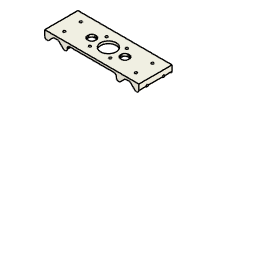
CHASSI_Pcb_SHELF (Autodesk Fusion 360 design; units mm, degrees)
Autodesk Fusion 360 part; units mm, degrees
note: some values were not read from the file. Set by a fixed rule: which sketch regions a step uses.
sketch "Sketch1" plane through (0, 21.15, 0) normal (0, 1, 0) x (-1, 0, 0)
  line L0 (-10, -11.15) -> (-10, 92)
  line L1 (-10, 92) -> (-12.5, 92)
  line L2 (-12.5, 92) -> (-12.5, -11.15)
  line L3 (-12.5, -11.15) -> (-10, -11.15)
  line L4 (112.5, -11.15) -> (112.5, 92)
  line L5 (112.5, 92) -> (110, 92)
  line L6 (110, 92) -> (110, -11.15)
  line L7 (110, -11.15) -> (112.5, -11.15)
  line L8 (81.2426, 69) -> (18.7574, 69)
  line L9 (18.7574, 69) -> (7.3788, 57.6216)
  line L10 (7.3788, 57.6216) -> (1.3788, 57.6216)
  line L11 (1.3788, 57.6216) -> (-10, 69.0007)
  line L12 (-10, 69.0007) -> (-10, 36.0007)
  line L13 (-10, 36.0007) -> (20, 66)
  line L14 (20, 66) -> (80, 66)
  line L15 (80, 66) -> (110, 36)
  line L16 (110, 36) -> (110, 69)
  line L17 (110, 69) -> (98.6213, 57.6213)
  line L18 (98.6213, 57.6213) -> (92.6213, 57.6213)
  line L19 (92.6213, 57.6213) -> (81.2426, 69)
  line L20 (50, 69) -> (50, 89) construction
  line L21 (-10, 92) -> (110, 92)
  line L22 (1.3788, 57.6216) -> (-10, 69.0007)
  line L23 (7.3788, 57.6216) -> (1.3788, 57.6216)
  line L24 (18.7574, 69) -> (7.3788, 57.6216)
  line L25 (4.3788, 57.6216) -> (4.3788, 89) construction
  line L26 (18.7574, 69) -> (7.3788, 57.6216)
  line L27 (7.3788, 57.6216) -> (1.3788, 57.6216)
  line L28 (1.3788, 57.6216) -> (-10, 69.0007)
  line L29 (7.3788, 57.6216) -> (18.7574, 69)
  line L30 (18.7574, 69) -> (24.7574, 69)
  line L31 (24.7574, 69) -> (36.1361, 57.621)
  line L32 (-9.9999, 77.6216) -> (1.3788, 89)
  line L33 (1.3788, 89) -> (7.3788, 89)
  line L34 (7.3788, 89) -> (18.7575, 77.621)
  line L35 (-10, 92) -> (-9.9999, 77.6216)
  line L36 (18.7575, 77.621) -> (18.7575, 89)
  line L37 (4.3788, 89) -> (7.3788, 89)
  line L38 (92.6213, 89) -> (81.2425, 77.621)
  line L39 (98.6213, 89) -> (92.6213, 89)
  line L40 (109.9999, 77.6216) -> (98.6213, 89)
  line L41 (81.2425, 77.621) -> (81.2425, 89)
  line L42 (18.7575, 89) -> (81.2425, 89)
  line L43 (92.6213, 89) -> (98.6213, 89)
  line L44 (110, 92) -> (109.9999, 77.6216)
  dimension "d70" = 20
  constraint midpoint L8 L20.start
  constraint perpendicular L8 L20
  constraint perpendicular L6 L37
  constraint midpoint L10 L25.start
  constraint perpendicular L25 L37
  constraint coincident L36.end L37
  constraint perpendicular L36 L37
  constraint collinear L37 L42
  constraint symmetric L20 L32.end L39.start
  constraint symmetric L20 L34.end L38.end
  constraint symmetric L20 L33.end L38.start
  constraint symmetric L20 L32.start L40.start
  constraint symmetric L20 L36.end L41.end
  constraint collinear L42 L43
  constraint coincident L5.end L6.start
  measures "d70" distance of L20.start L20.end
extrude "Extrude1" add sketch "Sketch1" against normal blind 42.3 contours L0 L6 L21 L32 L33 L34 L35 L36 L37 L38 L39 L40 L41 L42 L43 L44
sketch "Sketch2" plane through (9.9991, 0, -0.0001) normal (1, 0, -0.00001) x (0, 1, 0)
  line L0 (21.15, 77.6217) -> (21.15, 92.0001)
  line L1 (21.15, 92.0001) -> (-21.15, 92.0001)
  line L2 (-21.15, 92.0001) -> (-21.15, 77.6217)
  line L3 (-21.15, 77.6217) -> (21.15, 77.6217)
  line L4 (-21.15, 84.8109) -> (0, 84.8109) construction
  line L5 (0, 84.8109) -> (21.15, 84.8109) construction
  circle A0 centre (-10.575, 84.8109) radius 1.5
  circle A1 centre (10.575, 84.8109) radius 1.5
  dimension "d74" = 3
  dimension "d75" = 3
  constraint midpoint L2 L4.start
  constraint perpendicular L2 L4
  constraint midpoint L0 L5.end
  constraint perpendicular L0 L5
  constraint midpoint L4 A0.centre
  constraint midpoint L5 A1.centre
  measures "d74" diameter of A0
  measures "d75" diameter of A1
extrude "Extrude2" cut sketch "Sketch2" against normal blind 4 contours A0 | A1
sketch "Sketch4" plane through (-109.9992, 0, -0.0009) normal (-1, 0, -0.000008) x (0, -1, 0)
  line L0 (-21.15, 92.0009) -> (-21.15, 77.6226)
  line L1 (-21.15, 77.6226) -> (21.15, 77.6226)
  line L2 (21.15, 77.6226) -> (21.15, 92.0009)
  line L3 (21.15, 92.0009) -> (-21.15, 92.0009)
  ellipse E0 centre (10.575, 84.8107) end of major axis (9.075, 84.8107) minor radius 1.5
  ellipse E1 centre (-10.575, 84.8107) end of major axis (-12.075, 84.8107) minor radius 1.5
  ellipse E2 centre (0, 60.7499) end of major axis (-1.5, 60.7499) minor radius 1.5
  ellipse E3 centre (-10.575, 52.4999) end of major axis (-12.075, 52.4999) minor radius 1.5
  ellipse E4 centre (10.575, 52.4999) end of major axis (9.075, 52.4999) minor radius 1.5
  ellipse E5 centre (0, 44.2499) end of major axis (-1.5, 44.2499) minor radius 1.5
  ellipse E6 centre (15.5, 15.4999) end of major axis (14, 15.4999) minor radius 1.5
  ellipse E7 centre (-15.5, 15.4999) end of major axis (-17, 15.4999) minor radius 1.5
  ellipse E8 centre (-15.5, -15.5001) end of major axis (-17, -15.5001) minor radius 1.5
  ellipse E9 centre (15.5, -15.5001) end of major axis (14, -15.5001) minor radius 1.5
  ellipse E10 centre (0, -0.0001) end of major axis (-11, -0.0001) minor radius 11
  line L4 (21.15, 91.9999) -> (21.15, -11.1501)
  ellipse E11 centre (11.15, -11.1501) end of major axis (21.15, -11.1501) minor radius 10 (11.15, -21.1501) -> (21.15, -11.1501) ccw
  line L5 (11.15, -21.1501) -> (-11.15, -21.1501)
  ellipse E12 centre (-11.15, -11.1501) end of major axis (-21.15, -11.1501) minor radius 10 (-21.15, -11.1501) -> (-11.15, -21.1501) ccw
  line L6 (-21.15, -11.1501) -> (-21.15, 91.9999)
  line L7 (-21.15, 91.9999) -> (21.15, 91.9999)
extrude "Extrude4" cut sketch "Sketch4" against normal blind 4 contours E0 | E1
sketch "Sketch5" plane through (0, 0, 92) normal (0, 0, 1) x (-1, 0, 0)
  line L0 (-10, -21.15) -> (110, -21.15)
  line L1 (110, -21.15) -> (110, 21.15)
  line L2 (110, 21.15) -> (-10, 21.15)
  line L3 (-10, 21.15) -> (-10, -21.15)
  line L4 (42.085, 16.575) -> (42.085, 21.15)
  line L5 (42.085, 21.15) -> (18.7574, 21.15)
  line L6 (18.7574, 21.15) -> (18.7574, -21.15)
  line L7 (18.7574, -21.15) -> (81.2426, -21.15)
  line L8 (81.2426, -21.15) -> (81.2426, 21.15)
  line L9 (81.2426, 21.15) -> (57.915, 21.15)
  line L10 (57.915, 21.15) -> (57.915, 16.575)
  arc A0 (51.915, 10.575) -> (57.915, 16.575) centre (51.915, 16.575) ccw
  line L11 (51.915, 10.575) -> (48.085, 10.575)
  arc A1 (42.085, 16.575) -> (48.085, 10.575) centre (48.085, 16.575) ccw
  circle A2 centre (62.915, -10.575) radius 1.5
  circle A3 centre (62.915, 10.575) radius 1.5
  circle A4 centre (37.085, -10.575) radius 1.5
  circle A5 centre (37.085, 10.575) radius 1.5
  line L12 (-10, -21.15) -> (-9.9999, -21.15)
  line L13 (-9.9999, -21.15) -> (1.3788, -21.15)
  line L14 (1.3788, -21.15) -> (7.3788, -21.15)
  line L15 (7.3788, -21.15) -> (18.7575, -21.15)
  line L16 (18.7575, -21.15) -> (81.2425, -21.15)
  line L17 (81.2425, -21.15) -> (92.6213, -21.15)
  line L18 (92.6213, -21.15) -> (98.6213, -21.15)
  line L19 (98.6213, -21.15) -> (109.9999, -21.15)
  line L20 (109.9999, -21.15) -> (110, -21.15)
  line L21 (110, -21.15) -> (-10, -21.15)
  line L22 (95.6213, -21.15) -> (95.6213, 21.15) construction
  line L23 (4.3788, -21.15) -> (4.3788, 21.15) construction
  line L24 (37.085, 10.575) -> (4.3788, 10.575) construction
  line L25 (37.085, -10.575) -> (4.3788, -10.575) construction
  line L26 (50, -21.15) -> (50, 21.15) construction
  circle A6 centre (4.3788, 10.575) radius 1.5
  circle A7 centre (4.3788, -10.575) radius 1.5
  circle A8 centre (95.6212, 10.575) radius 1.5
  circle A9 centre (95.6212, -10.575) radius 1.5
  dimension "d86" = 3
  dimension "d87" = 3
  constraint midpoint L18 L22.start
  constraint coincident L2 L22.end
  constraint perpendicular L2 L22
  constraint midpoint L14 L23.start
  constraint coincident L2 L23.end
  constraint perpendicular L2 L23
  constraint coincident A5.centre L24.start
  constraint coincident L23 L24.end
  constraint perpendicular L23 L24
  constraint coincident A4.centre L25.start
  constraint coincident L23 L25.end
  constraint perpendicular L23 L25
  constraint midpoint L21 L26.start
  constraint midpoint L2 L26.end
  constraint coincident L24.end A6.centre
  constraint coincident L25.end A7.centre
  constraint symmetric L26 A6 A8
  constraint symmetric L26 A7 A9
  measures "d86" diameter of A6
  measures "d87" diameter of A7
extrude "Extrude5" cut sketch "Sketch5" against normal blind 3 contours A2 | A3 | A4 | A5 | A6 | A7 | A8 | A9
sketch "Sketch6" plane through (0, 0, 92) normal (0, 0, 1) x (-1, 0, 0)
  circle A0 centre (95.6212, 10.575) radius 1.5
  circle A1 centre (37.085, 10.575) radius 1.5
  circle A2 centre (62.915, 10.575) radius 1.5
  circle A3 centre (37.085, -10.575) radius 1.5
  circle A4 centre (62.915, -10.575) radius 1.5
  circle A5 centre (4.3788, 10.575) radius 1.5
  circle A6 centre (95.6212, -10.575) radius 1.5
  circle A7 centre (4.3788, -10.575) radius 1.5
  line L0 (-10, -21.15) -> (110, -21.15)
  line L1 (110, -21.15) -> (110, 21.15)
  line L2 (110, 21.15) -> (-10, 21.15)
  line L3 (-10, 21.15) -> (-10, -21.15)
  line L4 (50, 21.15) -> (50, -21.15) construction
  circle A8 centre (50, 0) radius 10
  line L5 (-10, 0) -> (110, 0) construction
  line L6 (37.085, 10.575) -> (4.3788, -10.575) construction
  line L7 (62.915, 10.575) -> (95.6212, -10.575) construction
  line L8 (20.7319, 0) -> (36.9872, 0) construction
  line L9 (29.8595, 5) -> (27.8595, 5)
  line L10 (23.8595, 1) -> (23.8595, -1)
  line L11 (27.8595, -5) -> (29.8595, -5)
  line L12 (33.8595, -1) -> (33.8595, 1)
  line L13 (33.8595, 5) -> (23.8595, -5) construction
  line L14 (23.8595, 5) -> (33.8595, -5) construction
  arc A9 (27.8595, 5) -> (23.8595, 1) centre (27.8595, 1) ccw
  arc A10 (23.8595, -1) -> (27.8595, -5) centre (27.8595, -1) ccw
  arc A11 (29.8595, -5) -> (33.8595, -1) centre (29.8595, -1) ccw
  arc A12 (33.8595, 1) -> (29.8595, 5) centre (29.8595, 1) ccw
  arc A13 (76.1405, 1) -> (72.1405, 5) centre (72.1405, 1) ccw
  line L15 (70.1405, 5) -> (72.1405, 5)
  arc A14 (70.1405, 5) -> (66.1405, 1) centre (70.1405, 1) ccw
  line L16 (66.1405, -1) -> (66.1405, 1)
  arc A15 (66.1405, -1) -> (70.1405, -5) centre (70.1405, -1) ccw
  line L17 (72.1405, -5) -> (70.1405, -5)
  arc A16 (72.1405, -5) -> (76.1405, -1) centre (72.1405, -1) ccw
  line L18 (76.1405, 1) -> (76.1405, -1)
  point P0 (28.8595, 0)
  dimension "d112" = 20
  dimension "d113" = 10
  dimension "d114" = 10
  dimension "d115" = 4
  constraint midpoint L2 L4.start
  constraint midpoint L0 L4.end
  constraint midpoint L4 A8.centre
  constraint midpoint L3 L5.start
  constraint midpoint L1 L5.end
  constraint coincident A1.centre L6.start
  constraint coincident A7.centre L6.end
  constraint coincident A2.centre L7.start
  constraint coincident A6.centre L7.end
  constraint midpoint L6 L8.start
  constraint coincident L5 L8.end
  constraint parallel L5 L8
  constraint horizontal L9
  constraint perpendicular L9 L10
  constraint parallel L9 L11
  constraint parallel L10 L12
  constraint coincident L13 P0
  constraint coincident L14 P0
  constraint midpoint L8 P0
  constraint coincident L14.start L9
  constraint coincident L14.start L10
  constraint tangent L9 A9
  constraint tangent L10 A9
  constraint coincident L13.end L10
  constraint coincident L13.end L11
  constraint tangent L10 A10
  constraint tangent L11 A10
  constraint equal A9 A10
  constraint coincident L14.end L11
  constraint coincident L14.end L12
  constraint tangent L11 A11
  constraint tangent L12 A11
  constraint equal A9 A11
  constraint coincident L13.start L12
  constraint coincident L13.start L9
  constraint tangent L12 A12
  constraint tangent L9 A12
  constraint equal A9 A12
  constraint symmetric L4 L9.end A13.end
  constraint symmetric L4 L10.start A13.start
  constraint symmetric L4 A9 A13
  constraint symmetric L4 L10.end A16.end
  constraint symmetric L4 L11.start L17.start
  constraint symmetric L4 A10 A16
  constraint symmetric L4 L11.end A15.end
  constraint symmetric L4 L12.start L16.start
  constraint symmetric L4 A11 A15
  constraint symmetric L4 L12.end A14.end
  constraint symmetric L4 L9.start L15.start
  constraint symmetric L4 A12 A14
  measures "d112" diameter of A8
  measures "d113" distance of L13.end L14.end
  measures "d114" distance of L14.start L13.end
  measures "d115" radius of A9
extrude "Extrude6" cut sketch "Sketch6" against normal up to surface (3 mm away) contours A8 | L9 L10 L11 L12 A9 A10 A11 A12 | A13 L15 A14 L16 A15 L17 A16 L18
fillet "Fillet1" radius 3 10 edges at (-98.6213, 0, 89) (-92.6213, 0, 89) (-109.9999, 0, 77.6216) (-81.2425, 0, 77.621) (-81.2425, 0, 89) (-18.7575, 0, 89) (-7.3788, 0, 89) (-18.7575, 0, 77.621) (-1.3788, 0, 89) (9.9999, 0, 77.6216)
